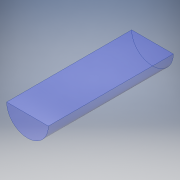
# Autodesk Inventor part: 00_Glassslab_Lens_Cylindrical_30mm_Plexiglas
Saved by Autodesk Inventor 2019 (Build 230136000, 136)
## iProperties
Created: 2021-02-03
Part Number: 00_Glassslab_Lens_Cylindrical_30mm_Plexiglas
Material: Glass
Document SubType Name: Modeling
Designer: diederichbenedict
Density: 2.18 g/cm^3
Appearance: Clear - Blue
Author: diederichbenedict
Autodesk Inventor part; units mm, degrees
ref_plane "YZ Plane" through (0, 0, 0) normal (1, 0, 0) x (0, 1, 0)
ref_plane "XZ Plane" through (0, 0, 0) normal (0, 1, 0) x (-1, 0, 0)
ref_plane "XY Plane" through (0, 0, 0) normal (0, 0, 1) x (1, 0, 0)
sketch "Sketch1" plane through (0, 0, 0) normal (0, 0, 1) x (1, 0, 0)
  line L0 (0, 0) -> (7.5, 0)
  line L1 (0, 0) -> (-7.5, 0)
  arc A0 (-7.5, 0) -> (7.5, 0) centre (0, 0) ccw
  dimension "d0" = 7.5
  dimension "d1" = 7.5
  dimension "d2" = 7.5
  constraints: 4 end point, 2 horizontal, 2 point on circle, 1 centre point
  measures "d0" distance of L0.start L0.end
  measures "d1" distance of L0.start L1.end
  measures "d2" radius of A0
extrude "Extrusion1" add sketch "Sketch1" along normal blind 45
body "Solid1"
